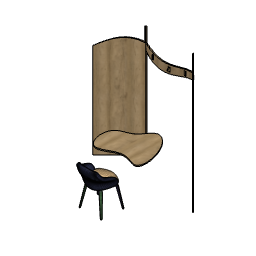
Installation v3 v3 (Autodesk Fusion 360 design; units mm, degrees)
Autodesk Fusion 360 part; units mm, degrees
sketch "Sketch1" plane through (0, 0, 0) normal (0, 1, 0) x (1, 0, 0) in component "Structure"
  line L0 (0, 0) -> (0, -1600)
  spline S0 degree 5 poles (-474.3629, -1805.3884) (-459.302, -1791.9355) (-428.8676, -1766.6681) (-382.2776, -1733.6822) (-318.2671, -1699.6033) (-235.1011, -1673.6504) (-148.9204, -1664.015) (-60.1245, -1669.4027) (30.4973, -1687.0242) (121.6054, -1711.924) (211.5229, -1737.8112) (298.4536, -1757.905) (380.706, -1765.7791) (456.9018, -1756.1442) (526.2714, -1725.925) (588.5292, -1673.8372) (632.634, -1614.4754) (662.5524, -1560.1191) (681.1035, -1519.5419) (690.0304, -1498.1684) knots 0 0 0 0 0 0 0.066667 0.133333 0.2 0.266667 0.333333 0.4 0.466667 0.533333 0.6 0.666667 0.733333 0.8 0.866667 0.933333 1 1 1 1 1 1
  spline S1 degree 5 poles (-473.0527, -1686.1641) (-461.1986, -1669.9659) (-436.806, -1639.454) (-398.1642, -1599.3396) (-342.5053, -1557.2441) (-266.0248, -1523.8368) (-182.9063, -1509.4746) (-93.9708, -1513.0694) (-0.827, -1532.1414) (93.7091, -1561.9774) (185.7688, -1595.8933) (271.0121, -1626.3168) (345.0773, -1645.5868) (404.0932, -1646.8546) (445.2237, -1625.0123) (467.2338, -1577.6443) (469.3388, -1518.7557) (462.2911, -1462.8539) (453.7864, -1420.4079) (448.5825, -1397.8904) knots 0 0 0 0 0 0 0.066667 0.133333 0.2 0.266667 0.333333 0.4 0.466667 0.533333 0.6 0.666667 0.733333 0.8 0.866667 0.933333 1 1 1 1 1 1
  line L1 (-54.9998, -1673.0419) -> (-53.3514, -1523.0419) construction
  line L2 (-474.3629, -1805.3884) -> (-473.0527, -1686.1641)
  line L3 (396.2541, -1760.7414) -> (397.5642, -1641.517)
  line L4 (-359.58, -1683.4551) -> (-329.58, -1683.4551)
  line L5 (-329.58, -1683.4551) -> (-329.58, -1603.4551)
  line L6 (-329.58, -1603.4551) -> (-359.58, -1603.4551)
  line L7 (-359.58, -1603.4551) -> (-359.58, -1683.4551)
  line L8 (-55.6454, -1638.9768) -> (-25.6454, -1638.9768)
  line L9 (-55.6454, -1558.9768) -> (-55.6454, -1638.9768)
  line L10 (-25.6454, -1638.9768) -> (-25.6454, -1558.9768)
  line L11 (-25.6454, -1558.9768) -> (-55.6454, -1558.9768)
  line L12 (244.0531, -1722.6383) -> (274.0531, -1722.6383)
  line L13 (244.0531, -1642.6383) -> (244.0531, -1722.6383)
  line L14 (274.0531, -1722.6383) -> (274.0531, -1642.6383)
  line L15 (274.0531, -1642.6383) -> (244.0531, -1642.6383)
  line L16 (-47.8549, -1627.9145) -> (-32.8549, -1627.9145)
  line L17 (-32.8549, -1627.9145) -> (-32.8549, -1597.9145)
  line L18 (-32.8549, -1597.9145) -> (-47.8549, -1597.9145)
  line L19 (-47.8549, -1597.9145) -> (-47.8549, -1627.9145)
  spline S2 degree 5 poles (690.0304, -1498.1684) (700.5111, -1475.7097) (720.4396, -1432.5307) (747.2348, -1372.977) (778.0901, -1304.2419) (815.7848, -1237.5602) (861.2343, -1191.8132) (922.2678, -1168.2614) (1002.895, -1166.3731) (1104.0459, -1184.4196) (1225.1762, -1220.4436) (1337.1348, -1262.2743) (1429.1118, -1300.4663) (1493.9303, -1328.9086) (1527.2148, -1343.875) knots 0 0 0 0 0 0 0.1 0.2 0.3 0.4 0.5 0.6 0.7 0.8 0.9 1 1 1 1 1 1
  line L20 (630.0274, -1626.7462) -> (750.0334, -1369.5906)
  line L21 (1527.2148, -1343.875) -> (1604.3615, -1218.1545)
  spline S3 degree 5 poles (-474.3629, -1805.3884) (-490.9177, -1821.0593) (-524.3372, -1849.0748) (-575.3956, -1881.1201) (-645.3451, -1903.7371) (-736.0617, -1898.6086) (-830.3914, -1861.822) (-928.9026, -1798.4534) (-1032.3929, -1717.3136) (-1141.7718, -1629.0718) (-1257.9545, -1544.9966) (-1381.7396, -1475.5548) (-1513.6538, -1428.9556) (-1653.8186, -1409.9199) (-1802.1216, -1420.7961) (-1958.3285, -1462.2942) (-2089.4134, -1519.8287) (-2191.0799, -1576.4323) (-2260.337, -1620.1038) (-2295.3354, -1643.4235) knots 0 0 0 0 0 0 0.066667 0.133333 0.2 0.266667 0.333333 0.4 0.466667 0.533333 0.6 0.666667 0.733333 0.8 0.866667 0.933333 1 1 1 1 1 1
  line L22 (1527.2148, -1343.875) -> (1527.2148, -2764.644)
  line L23 (1527.2148, -2764.644) -> (-27.9454, -2764.644)
  line L24 (-27.9454, -2764.644) -> (396.2541, -1760.7414)
  line L25 (-474.3629, -1805.3884) -> (-175.3904, -2753.6089)
  line L26 (-175.3904, -2753.6089) -> (-2314.6316, -2677.1006)
  line L27 (-2314.6316, -2677.1006) -> (-2295.3354, -1643.4235)
  point P0 (-474.3629, -1805.3884)
  point P1 (-54.9998, -1673.0419)
  point P2 (396.2541, -1760.7414)
  point P3 (-54.9998, -1673.0419)
  point P4 (396.2541, -1760.7414)
  point P5 (-473.0527, -1686.1641)
  point P6 (-53.3514, -1523.0419)
  point P7 (397.5642, -1641.517)
  point P8 (1.3102, -1480.7757)
  point P9 (397.5642, -1641.517)
  point P10 (-53.3514, -1523.0419)
  point P11 (878.6112, -1189.5816)
  point P12 (-795.261, -1872.0062)
  point P13 (-1366.718, -1489.1301)
  point P14 (-335.1889, -2246.7923)
  point P15 (215.0156, -2189.6569)
  dimension "d1" = 1600
  dimension "d2" = 150
  dimension "d5" = 30
  dimension "d6" = 80
  dimension "d7" = 30
  dimension "d8" = 80
  dimension "d9" = 30
  dimension "d10" = 80
  dimension "d14" = 15
  dimension "d15" = 30
  constraint coincident L0.start origin
  constraint vertical L0
  constraint coincident P3 P1
  constraint coincident P4 P2
  constraint coincident P10 P6
  constraint coincident P9 P7
  constraint parallel L1 L3
  constraint horizontal L4
  constraint vertical L5
  constraint horizontal L6
  constraint vertical L7
  constraint horizontal L8
  constraint vertical L10
  constraint horizontal L11
  constraint vertical L9
  constraint horizontal L12
  constraint vertical L14
  constraint horizontal L15
  constraint vertical L13
  constraint horizontal L16
  constraint vertical L17
  constraint horizontal L18
  constraint vertical L19
  constraint midpoint S0.end L20
  constraint coincident P0 S0.start
  constraint vertical L22
  constraint perpendicular L22 L23
  constraint coincident L25 P14
  constraint coincident L24 P15
  measures "d1" distance of L0.start L0.end
  measures "d2" vertical distance of P3 P10
  measures "d5" distance of L4.start L4.end
  measures "d6" distance of L4.start L6.end
  measures "d7" distance of L8.end L8.start
  measures "d8" distance of L8.start L9.start
  measures "d9" distance of L12.end L12.start
  measures "d10" distance of L12.start L13.start
  measures "d14" distance of L16.start L16.end
  measures "d15" distance of L16.start L18.end
extrude "Extrude1" add sketch "Sketch1" along normal blind 20 contours S0 S1 L2 L3 | L4 L5 L6 L7 | L8 L9 L10 L11 | L12 L13 L14 L15 | L16 L17 L18 L19 makes body 1 in component "Structure"
extrude "Extrude2" cut sketch "Sketch1" along normal blind 100 contours L4 L5 L6 L7 | L8 L9 L10 L11 | L12 L13 L14 L15 | L16 L17 L18 L19 bodies 1 in component "Structure"
revolve "Revolve1" add sketch "Sketch1" angle 360 about axis through (-32.8549, 0, 1597.9145) along (-1, 0, 0) separate body contours L16 L17 L18 L19 makes body 2 in component "Structure"
sketch "Sketch2" plane through (0, 0, 0) normal (0, 0, 1) x (1, 0, 0) in component "Structure"
  line L0 (-474.3629, 0) -> (396.2541, 0)
  line L1 (396.2541, 0) -> (396.2541, 20)
  line L2 (-474.3629, 20) -> (396.2541, 20)
  line L3 (-474.3629, 20) -> (-474.3629, 0)
  line L4 (396.2541, 0) -> (891.2288, -494.9747)
  line L5 (396.2541, 0) -> (1096.2541, 0) construction
  line L6 (396.2541, 20) -> (901.2288, -484.9747)
  line L7 (891.2288, -494.9747) -> (901.2288, -484.9747)
  line L8 (-474.3629, 0) -> (-969.3376, -494.9747)
  line L9 (-474.3629, 0) -> (225.6371, 0) construction
  line L10 (-474.3629, 20) -> (-979.3376, -484.9747)
  line L11 (-979.3376, -484.9747) -> (-969.3376, -494.9747)
  dimension "d17" = 45
  dimension "d18" = 700
  dimension "d19" = 135
  dimension "d20" = 700
  constraint horizontal L5
  constraint coincident L0.end L1.start
  constraint coincident L1.end L2.end
  constraint parallel L4 L6
  constraint perpendicular L4 L7
  constraint horizontal L9
  constraint coincident L0.start L3.end
  constraint coincident L2.start L3.start
  constraint parallel L8 L10
  constraint perpendicular L8 L11
  measures "d17" angle of L4 L5
  measures "d18" distance of L0.end L4.end
  measures "d19" angle of L8 L9
  measures "d20" distance of L0.start L8.end
extrude "Extrude3" add sketch "Sketch2" along normal blind 2073.423 contours L3 L8 L10 L11 | L1 L4 L6 L7 bodies 1 in component "Structure"
extrude "Extrude5" cut sketch "Sketch1" against normal blind 1621.85 contours S0 S2 L22 L23 L24 | S3 L25 L26 L27 bodies 1 in component "Structure"
sketch "Sketch3" plane through (0, 0, 0) normal (0, 0, 1) x (1, 0, 0) in component "Structure"
  spline S0 degree 5 poles (-208.5679, -491.2858) (-197.6683, -483.8235) (-176.8011, -467.748) (-148.3841, -440.0119) (-115.5128, -396.811) (-77.6262, -340.686) (-36.819, -293.3991) (11.9309, -265.9157) (69.8497, -265.9451) (134.3319, -296.9855) (200.5336, -358.8281) (262.4956, -447.5469) (314.3717, -555.7891) (351.8158, -672.6289) (372.2186, -785.1039) (374.3737, -880.5369) (358.3353, -948.567) (325.207, -983.4052) (276.9646, -985.8027) (216.2822, -965.7574) (146.2473, -938.706) (70.0459, -920.5612) (-9.3177, -923.479) (-89.3668, -950.5736) (-168.3073, -993.3387) (-244.5962, -1037.1547) (-316.6189, -1065.3206) (-382.3127, -1063.725) (-438.8394, -1025.0766) (-482.1578, -953.8294) (-507.9665, -862.3404) (-512.7082, -766.5295) (-494.6309, -681.5469) (-454.6673, -617.8952) (-397.8377, -576.1792) (-332.0397, -548.8929) (-279.0034, -529.8999) (-242.1986, -512.5218) (-219.4675, -498.7481) (-208.5679, -491.2858) knots 0 0 0 0 0 0 0.028571 0.057143 0.085714 0.114286 0.142857 0.171429 0.2 0.228571 0.257143 0.285714 0.314286 0.342857 0.371429 0.4 0.428571 0.457143 0.485714 0.514286 0.542857 0.571429 0.6 0.628571 0.657143 0.685714 0.714286 0.742857 0.771429 0.8 0.828571 0.857143 0.885714 0.914286 0.942857 0.971429 1 1 1 1 1 1
  point P0 (-16.7383, -285.6128)
  point P1 (277.9279, -485.3529)
  point P2 (315.5028, -977.7815)
  point P3 (10.9485, -926.3633)
  point P4 (-384.5765, -1052.9313)
  point P5 (-479.5025, -665.3168)
extrude "Extrude6" add sketch "Sketch3" along normal blind 20 from surface at 700 separate body makes body 3 in component "Structure"
other "Base Mesh Feature1" in component "Structure"
component "Structure" placed x (1, 0, 0) y (0, 1, 0) z (0, 0, 1) at (0, 0, 0)
